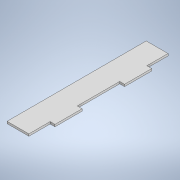
# Autodesk Inventor part: track_guides_3mm
Saved by Autodesk Inventor 2021 (Build 250183000, 183)
## iProperties
Created: 2021-02-11
Part Number: track_guides_3mm
Material: Generic
Document SubType Name: Modeling
Designer: apat475
Density: 1 g/cm^3
Appearance: Default
Author: apat475
Autodesk Inventor part; units mm, degrees
ref_plane "YZ Plane" through (0, 0, 0) normal (1, 0, 0) x (0, 1, 0)
ref_plane "XZ Plane" through (0, 0, 0) normal (0, 1, 0) x (-1, 0, 0)
ref_plane "XY Plane" through (0, 0, 0) normal (0, 0, 1) x (1, 0, 0)
sketch "Sketch1" plane through (0, 0, 0) normal (0, 1, 0) x (-1, 0, 0)
  line L0 (40.8683, 149.0264) -> (9.5242, 149.0264)
  line L1 (9.5242, -50.9736) -> (40.8683, -50.9736)
  line L2 (40.8683, -50.9736) -> (40.8683, 149.0264)
  line L3 (9.5242, 118.5264) -> (2.5242, 118.5264)
  line L4 (2.5242, 118.5264) -> (2.5242, 79.5264)
  line L5 (2.5242, 79.5264) -> (9.5242, 79.5264)
  line L6 (9.5242, 18.5264) -> (2.5242, 18.5264)
  line L7 (2.5242, 18.5264) -> (2.5242, -20.4736)
  line L8 (2.5242, -20.4736) -> (9.5242, -20.4736)
  line L9 (9.5242, 149.0264) -> (9.5242, 118.5264)
  line L10 (9.5242, 79.5264) -> (9.5242, 18.5264)
  line L11 (9.5242, -20.4736) -> (9.5242, -50.9736)
  point P0 (0, 0)
  dimension "d1" = 200
  dimension "d2" = 30.5
  dimension "d3" = 30.5
  dimension "d4" = 61
  dimension "d5" = 39
  dimension "d6" = 7
  constraints: 24 end point, 8 parallel, 5 perpendicular, 3 horizontal, 1 point on line
  measures "d1" distance of L1.end L0.start
  measures "d2" distance between parallel lines of L0 L3
  measures "d3" distance between parallel lines of L8 L1
  measures "d4" distance of L5.end L6.start
  measures "d5" distance of L3.end L4.end
  measures "d6" distance of L3.start L3.end
extrude "Extrusion1" add sketch "Sketch1" along normal blind 3
body "Solid1"
